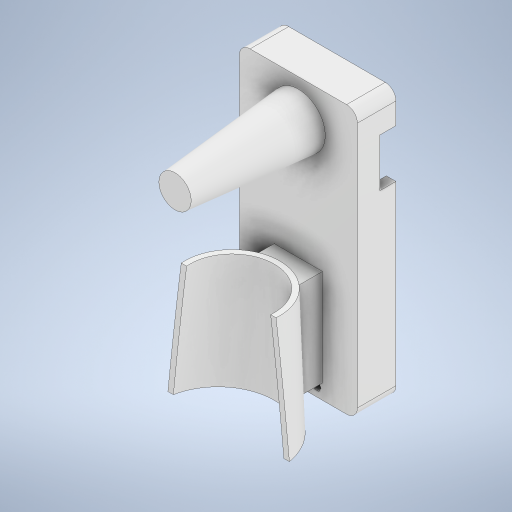
# Autodesk Inventor part: hand_rest_v4
Saved by Autodesk Inventor 2024 (Build 280153000, 153)
## iProperties
Created: 2023-07-30
Part Number: hand_rest_v4
Material: ABS Plastic
Document SubType Name: Modeling
Designer: Pintu
Density: 1.06 g/cm^3
Appearance: Smooth - White
Author: Pintu
Autodesk Inventor part; units mm, degrees
ref_plane "YZ Plane" through (0, 0, 0) normal (1, 0, 0) x (0, 1, 0)
ref_plane "XY Plane" through (0, 0, 0) normal (0, 0, 1) x (1, 0, 0)
sketch "Sketch1" plane through (0, 0, 0) normal (0, 0, 1) x (1, 0, 0)
  line L0 (-55, 125) -> (55, 125)
  line L1 (55, 125) -> (55, -125)
  line L2 (55, -125) -> (-55, -125)
  line L3 (-55, -125) -> (-55, 125)
  line L4 (-55, 125) -> (55, -125) construction
  line L5 (55, 125) -> (-55, -125) construction
  point P0 (0, 0)
  dimension "d0" = 110
  dimension "d1" = 250
  constraints: 12 end point, 2 midpoint, 2 parallel, 1 horizontal, 1 perpendicular
  measures "d0" distance of L1.end L2.end
  measures "d1" distance of L0.end L1.end
extrude "Extrusion1" add sketch "Sketch1" along normal blind 6
fillet "Fillet1" radius 10 4 edges at (-55, 125, 3) (55, 125, 3) (-55, -125, 3) (55, -125, 3)
sketch "Sketch2" plane through (0, 0, 6) normal (0, 0, 1) x (1, 0, 0)
  line L0 (-45, -125) -> (45, -125) projected
  point P0 (0, 0)
  point P1 (0.0434, -121)
  dimension "d5" = 4
  measures "d5" distance from line of L0 point (0.043, -121)
hole "Hole1" at (0.0434, -121, 6) direction (0, 0, -1) diameter 3 end through all
sketch "Sketch4" plane through (0, 0, 0) normal (0, 1, 0) x (-1, 0, 0)
  line L0 (-1.5434, 6) -> (1.4566, 6) projected
  line L1 (-55, 6) -> (-45, 6) projected
  line L2 (-45, 6) -> (-55, 6) projected
  line L3 (-45, 6) -> (45, 6) projected
  line L4 (55, 6) -> (45, 6) projected
  line L5 (45, 6) -> (55, 6) projected
  line L6 (45, 6) -> (-45, 6) projected
  circle A0 centre (0, 66) radius 42.5
  circle A1 centre (0, 66) radius 37.5
  point P0 (0, 0)
  point P1 (0, 6)
  dimension "frontOuterDia" = 85
  dimension "d17" = 60
  dimension "frontInnerDia" = 75
  constraints: 2 centre point, 1 coincident, 1 midpoint
  measures "frontOuterDia" diameter of A0
  measures "d17" distance of point (0, 6) A0.centre
  measures "frontInnerDia" diameter of A1
sketch "Sketch3" plane through (-45, -125, 0) normal (0, -1, 0) x (1, 0, 0)
  line L0 (0, 6) -> (90, 6) projected
  circle A0 centre (45, 81) radius 57.5
  circle A1 centre (45, 81) radius 52.5
  point P0 (45, 0)
  point P1 (45, 6)
  dimension "outerDia" = 115
  dimension "restHeight" = 75
  dimension "innerRearDia" = 105
  constraints: 2 centre point, 1 coincident, 1 midpoint
  measures "outerDia" diameter of A0
  measures "restHeight" distance of point (45, 6) A0.centre
  measures "innerRearDia" diameter of A1
loft "Loft1" add profiles "Sketch3", "Sketch4" contours A0 | A1 / A0 | A1
loft "Loft2" cut profiles "Sketch3", "Sketch4" contours A1 / A1
sketch "Sketch5" plane through (0, 0, 6) normal (0, 0, 1) x (1, 0, 0)
  line L0 (-22.5, -21) -> (22.5, -21)
  line L1 (22.5, -21) -> (22.5, -111)
  line L2 (22.5, -111) -> (-22.5, -111)
  line L3 (-22.5, -111) -> (-22.5, -21)
  line L4 (-22.5, -21) -> (22.5, -111) construction
  line L5 (22.5, -21) -> (-22.5, -111) construction
  line L6 (-45, -125) -> (45, -125) projected
  point P0 (0, 0)
  point P1 (0, -66)
  dimension "d27" = 45
  dimension "d28" = 90
  dimension "d142" = 14
  constraints: 12 end point, 2 midpoint, 2 parallel, 1 horizontal, 1 perpendicular
  measures "d27" distance of L1.end L2.end
  measures "d28" distance of L0.end L1.end
  measures "d142" distance between parallel lines of L6 L2
extrude "Extrusion2" add sketch "Sketch5" along normal blind 22
sketch "Sketch6" plane through (0, 0, 6) normal (0, 0, 1) x (1, 0, 0)
  circle A0 centre (0, 90) radius 25
  line L0 (45, 125) -> (-45, 125) projected
  line L1 (55, -115) -> (55, 115) projected
  point P0 (0, 0)
  dimension "d34" = 50
  dimension "d35" = 35
  dimension "d36" = 55
  constraints: 1 centre point
  measures "d34" diameter of A0
  measures "d35" distance from line of L0 A0.centre
  measures "d36" distance from line of L1 A0.centre
ref_plane "Work Plane3" through (0, 0, 121) normal (0, 0, 1) x (1, 0, 0)
sketch "Sketch7" plane through (0, 0, 121) normal (0, 0, 1) x (1, 0, 0)
  line L0 (45, 125) -> (-45, 125) projected
  circle A0 centre (0, 90) radius 15
  point P0 (0, 0)
  point P1 (0, 125)
  dimension "d38" = 30
  dimension "d39" = 35
  constraints: 1 centre point, 1 midpoint
  measures "d38" diameter of A0
  measures "d39" distance of point (0, 125) A0.centre
loft "Loft3" add profiles "Sketch6", "Sketch7"
ref_plane "Work Plane4" through (0, 0, 71) normal (0, 0, 1) x (1, 0, 0)
sketch "Sketch9" plane through (0, 0, 71) normal (0, 0, 1) x (1, 0, 0)
  line L0 (78.1064, 17.385) -> (-78.1064, 17.385)
  line L1 (-78.1064, 17.385) -> (-78.1064, -125.7261)
  line L2 (-78.1064, -125.7261) -> (78.1064, -125.7261)
  line L3 (78.1064, -125.7261) -> (78.1064, 17.385)
  line L4 (78.1064, 17.385) -> (-78.1064, -125.7261) construction
  line L5 (-78.1064, 17.385) -> (78.1064, -125.7261) construction
  point P0 (0, 0)
  point P1 (0, -54.1705)
  constraints: 12 end point, 2 midpoint, 2 parallel, 1 horizontal, 1 perpendicular
extrude "Extrusion4" cut sketch "Sketch9" along normal blind 100
ref_plane "Work Plane5" through (0, -15, 0) normal (0, 1, 0) x (-1, 0, 0)
sketch "Sketch19" plane through (0, -15, 0) normal (0, 1, 0) x (-1, 0, 0)
  point P0 (0, 0)
sketch "Sketch20" plane through (0, 0, 6) normal (0, 0, 1) x (1, 0, 0)
  line L0 (-80.5, -15) -> (80.5, -15) projected
  line L1 (55, -115) -> (55, 115) projected
  line L2 (-55, 115) -> (-55, -115) projected
  line L3 (55, -15) -> (-55, -15)
  line L4 (-55, -15) -> (-55, 0)
  line L5 (-55, 0) -> (55, 0)
  line L6 (55, 0) -> (55, -15)
  point P0 (0, 0)
  constraints: 8 end point, 2 parallel, 2 point on line, 1 horizontal, 1 midpoint, 1 perpendicular
extrude "Extrusion5" cut sketch "Sketch20" along normal blind 99.75
sketch "Sketch22" plane through (0, 0, 0) normal (0, 0, -1) x (-1, 0, 0)
  line L0 (55, 115) -> (55, -115) projected
  arc A0 (55, 115) -> (45, 125) centre (45, 115) ccw projected
  line L1 (-45, 125) -> (45, 125) projected
  arc A1 (-45, 125) -> (-55, 115) centre (-45, 115) ccw projected
  line L2 (-55, -115) -> (-55, 115) projected
  arc A2 (-55, -115) -> (-45, -125) centre (-45, -115) ccw projected
  line L3 (45, -125) -> (-45, -125) projected
  arc A3 (45, -125) -> (55, -115) centre (45, -115) ccw projected
  line L4 (46, -115) -> (46, 115)
  arc A4 (46, 115) -> (45, 116) centre (45, 115) ccw
  line L5 (45, 116) -> (-45, 116)
  arc A5 (-45, 116) -> (-46, 115) centre (-45, 115) ccw
  line L6 (-46, 115) -> (-46, -115)
  arc A6 (-46, -115) -> (-45, -116) centre (-45, -115) ccw
  line L7 (-45, -116) -> (45, -116)
  arc A7 (45, -116) -> (46, -115) centre (45, -115) ccw
  line L8 (-55, 95) -> (-37, 95)
  line L9 (-37, 95) -> (-37, 50)
  line L10 (-37, 50) -> (-55, 50)
  line L11 (-55, 50) -> (-55, 95)
  line L12 (0, -177.9853) -> (0, 178.4142) projected
  line L13 (22.5, -107) -> (-22.5, -107)
  line L14 (-22.5, -107) -> (-22.5, -125)
  line L15 (-22.5, -125) -> (22.5, -125)
  line L16 (22.5, -125) -> (22.5, -107)
  line L17 (22.5, -107) -> (-22.5, -125) construction
  line L18 (-22.5, -107) -> (22.5, -125) construction
  line L19 (55, 95) -> (37, 95)
  line L20 (37, 95) -> (37, 50)
  line L21 (37, 50) -> (55, 50)
  line L22 (55, 50) -> (55, 95)
  point P0 (0, 0)
  point P1 (0, -116)
  point P2 (-46, 95)
  point P3 (46, 95)
  point P4 (-22.5, -116)
  point P5 (-46, 50)
  point P6 (-55, 50)
  point P7 (46, 50)
  point P8 (22.5, -116)
  dimension "d146" = 9
  dimension "d147" = 18
  dimension "d148" = 45
  dimension "d149" = 30
  dimension "d150" = 45
  dimension "d151" = 18
  dimension "d152" = 0
  dimension "d153" = 18
  dimension "d154" = 45
  dimension "d155" = 30
  constraints: 36 end point, 8 point on circle, 6 parallel, 4 centre point, 3 horizontal, 3 perpendicular, 3 point on line, 2 midpoint, 7 other
  measures "d146" distance between parallel lines of L0 L4
  measures "d147" distance of L9.end L10.end
  measures "d148" distance of L8.end L9.end
  measures "d149" distance between parallel lines of L1 L8
  measures "d150" distance of L15.end L14.end
  measures "d151" distance of L14.end L13.end
  measures "d152" distance between parallel lines of L3 L15
  measures "d153" distance of L21.end L20.end
  measures "d154" distance of L20.end L19.end
  measures "d155" distance between parallel lines of L1 L19
extrude "Extrusion6" add sketch "Sketch22" along normal blind 30 contours L0 L19 L4 A4 L5 L12 L1 A0 | L0 A3 L3 L16 L7 A7 L4 L21 | L12 L5 A5 L6 L8 L2 A1 L1 | L10 L6 A6 L7 L14 L3 A2 L2
sketch "Sketch26" plane through (0, 0, 0) normal (0, 0, -1) x (-1, 0, 0)
  line L0 (-55, 115) -> (-55, 95) projected
  line L1 (-55, 95) -> (-46, 95) projected
  line L2 (-46, 95) -> (-46, 115) projected
  arc A0 (-45, 116) -> (-46, 115) centre (-45, 115) ccw projected
  line L3 (-45, 116) -> (45, 116) projected
  arc A1 (46, 115) -> (45, 116) centre (45, 115) ccw projected
  line L4 (46, 115) -> (46, 95) projected
  line L5 (46, 95) -> (55, 95) projected
  line L6 (55, 95) -> (55, 115) projected
  arc A2 (55, 115) -> (45, 125) centre (45, 115) ccw projected
  line L7 (45, 125) -> (-45, 125) projected
  arc A3 (-45, 125) -> (-55, 115) centre (-45, 115) ccw projected
  line L8 (46, 50) -> (46, -115) projected
  line L9 (55, -115) -> (55, 50) projected
  line L10 (55, 50) -> (46, 50) projected
  line L11 (46, 50) -> (46, -115) projected
  arc A4 (45, -116) -> (46, -115) centre (45, -115) ccw projected
  line L12 (45, -116) -> (22.5, -116) projected
  line L13 (22.5, -116) -> (22.5, -125) projected
  line L14 (22.5, -125) -> (45, -125) projected
  arc A5 (45, -125) -> (55, -115) centre (45, -115) ccw projected
  line L15 (-45, -125) -> (-22.5, -125) projected
  line L16 (-22.5, -125) -> (-22.5, -116) projected
  line L17 (-22.5, -116) -> (-45, -116) projected
  arc A6 (-46, -115) -> (-45, -116) centre (-45, -115) ccw projected
  line L18 (-46, -115) -> (-46, 50) projected
  line L19 (-46, 50) -> (-55, 50) projected
  line L20 (-55, 50) -> (-55, -115) projected
  arc A7 (-55, -115) -> (-45, -125) centre (-45, -115) ccw projected
  line L21 (-55, 95) -> (-37, 95)
  line L22 (-37, 95) -> (-37, 50)
  line L23 (-37, 50) -> (-55, 50)
  line L24 (-55, 50) -> (-55, 95)
  line L25 (-46, 50) -> (-55, 50) projected
  point P0 (0, 0)
  dimension "d168" = 18
  constraints: 8 end point, 2 parallel, 1 collinear, 1 horizontal, 1 perpendicular
  measures "d168" distance of L22.end L23.end
extrude "Extrusion8" add sketch "Sketch26" along normal blind 15 contours L1 L21 L22 L23 L19 L24
ref_plane "Work Plane6" through (46, 49, 0) normal (-1, 0, 0) x (0, 0, 1)
sketch "Sketch29" plane through (46, 49, 0) normal (-1, 0, 0) x (0, 0, 1)
  line L0 (-15, 46) -> (-15, 1) projected
  circle A0 centre (-15, 23.5) radius 11.5
  point P0 (0, -49)
  dimension "d171" = 23
  constraints: 1 centre point, 1 midpoint
  measures "d171" diameter of A0
extrude "Extrusion9" cut sketch "Sketch29" along normal mid plane 7
sketch "Sketch30" plane through (0, 0, 0) normal (0, 0, -1) x (-1, 0, 0)
  line L0 (-55, 115) -> (-55, 95) projected
  line L1 (-55, 95) -> (-46, 95) projected
  line L2 (-46, 95) -> (-46, 115) projected
  arc A0 (-45, 116) -> (-46, 115) centre (-45, 115) ccw projected
  line L3 (-45, 116) -> (45, 116) projected
  arc A1 (46, 115) -> (45, 116) centre (45, 115) ccw projected
  line L4 (46, 115) -> (46, 95) projected
  line L5 (46, 95) -> (55, 95) projected
  line L6 (55, 95) -> (55, 115) projected
  arc A2 (55, 115) -> (45, 125) centre (45, 115) ccw projected
  line L7 (45, 125) -> (-45, 125) projected
  arc A3 (-45, 125) -> (-55, 115) centre (-45, 115) ccw projected
  line L8 (55, -115) -> (55, 50) projected
  line L9 (55, 50) -> (46, 50) projected
  line L10 (46, 50) -> (46, -115) projected
  arc A4 (45, -116) -> (46, -115) centre (45, -115) ccw projected
  line L11 (45, -116) -> (22.5, -116) projected
  line L12 (22.5, -116) -> (22.5, -125) projected
  line L13 (22.5, -125) -> (45, -125) projected
  arc A5 (45, -125) -> (55, -115) centre (45, -115) ccw projected
  line L14 (-45, -125) -> (-22.5, -125) projected
  line L15 (-22.5, -125) -> (-22.5, -116) projected
  line L16 (-22.5, -116) -> (-45, -116) projected
  arc A6 (-46, -115) -> (-45, -116) centre (-45, -115) ccw projected
  line L17 (-46, -115) -> (-46, 50) projected
  line L18 (-46, 50) -> (-55, 50) projected
  line L19 (-55, 50) -> (-55, -115) projected
  arc A7 (-55, -115) -> (-45, -125) centre (-45, -115) ccw projected
  line L20 (55, 95) -> (55, 50) projected
  line L21 (55, 95) -> (37, 95)
  line L22 (37, 95) -> (37, 50)
  line L23 (37, 50) -> (55, 50)
  line L24 (55, 50) -> (55, 95)
  line L25 (-22.5, -125) -> (22.5, -125)
  line L26 (22.5, -125) -> (22.5, -107)
  line L27 (22.5, -107) -> (-22.5, -107)
  line L28 (-22.5, -107) -> (-22.5, -125)
  point P0 (0, 0)
  dimension "d174" = 18
  dimension "d175" = 18
  constraints: 16 end point, 4 parallel, 2 horizontal, 2 perpendicular, 1 point on line
  measures "d174" distance between parallel lines of L20 L22
  measures "d175" distance of L26.end L25.end
extrude "Extrusion10" add sketch "Sketch30" along normal blind 15 contours L20 L9 L23 L22 L21 L5 | L25 L15 L28 L27 L26 L12
ref_plane "Work Plane7" through (-46, -115, 6) normal (-1, 0, 0) x (0, 0, 1)
sketch "Sketch31" plane through (-46, -115, 6) normal (-1, 0, 0) x (0, 0, 1)
  line L0 (-21, 176) -> (-21, 199) projected
  circle A0 centre (-21, 187.5) radius 11.5
  point P0 (-6, 115)
  dimension "d178" = 23
  constraints: 1 centre point, 1 midpoint
  measures "d178" diameter of A0
extrude "Extrusion11" cut sketch "Sketch31" along normal mid plane 7
ref_plane "Work Plane9" through (-22.5, -116, 0) normal (0, 1, 0) x (1, 0, 0)
sketch "Sketch33" plane through (-22.5, -116, 0) normal (0, 1, 0) x (1, 0, 0)
  line L0 (45, 15) -> (0, 15) projected
  circle A0 centre (22.5, 15) radius 11.5
  point P0 (22.5, 0)
  dimension "d182" = 23
  constraints: 1 centre point, 1 midpoint
  measures "d182" diameter of A0
extrude "Extrusion12" cut sketch "Sketch33" along normal mid plane 7
fillet "Fillet15" radius 3 6 edges at (37, 50, -7.5) (37, 95, -7.5) (-37, 95, -7.5) (-37, 50, -7.5) (22.5, -107, -7.5) (-22.5, -107, -7.5) inverted yes
fillet "Fillet16" radius 2 12 edges at (19.5, -107, -7.5) (22.5, -110, -7.5) (-19.5, -107, -7.5) (-22.5, -110, -7.5) (37, 53, -7.5) (40, 50, -7.5) (37, 92, -7.5) (40, 95, -7.5) (-37, 92, -7.5) (-40, 95, -7.5) (-37, 53, -7.5) (-40, 50, -7.5)
sketch "Sketch45" plane through (0, 0, -15) normal (0, 0, -1) x (-1, 0, 0)
  line L0 (11.5, -112.5) -> (11.5, -119.5) projected
  line L1 (-22.5, -125) -> (22.5, -125) projected
  point P0 (0, 0)
  point P1 (17, -116)
  dimension "d236" = 5.5
  dimension "d237" = 9
  measures "d236" distance from line of L0 point (17, -116)
  measures "d237" distance from line of L1 point (17, -116)
hole "Hole12" at (-17, -116, -15) direction (0, 0, 1) diameter 4 depth 25 tip angle 118
sketch "Sketch46" plane through (0, 0, -15) normal (0, 0, -1) x (-1, 0, 0)
  line L0 (-11.5, -119.5) -> (-11.5, -112.5) projected
  line L1 (-22.5, -125) -> (22.5, -125) projected
  point P0 (0, 0)
  point P1 (-17, -116)
  dimension "d245" = 5.5
  dimension "d246" = 9
  measures "d245" distance from line of L0 point (-17, -116)
  measures "d246" distance from line of L1 point (-17, -116)
hole "Hole13" at (17, -116, -15) direction (0, 0, 1) diameter 4 depth 25 tip angle 118
sketch "Sketch47" plane through (0, 0, 6) normal (0, 0, 1) x (1, 0, 0)
  circle A0 centre (17, -116) radius 2 projected
  circle A1 centre (-17, -116) radius 2 projected
  line L0 (-11.5, -119.5) -> (11.5, -119.5) projected
  line L1 (11.5, -119.5) -> (11.5, -112.5) projected
  line L2 (11.5, -112.5) -> (-11.5, -112.5) projected
  line L3 (-11.5, -112.5) -> (-11.5, -119.5) projected
  arc A2 (-21.3, -109.7495) -> (-22.5, -111.5826) centre (-20.5, -111.5826) ccw projected
  arc A3 (-21.3, -109.7495) -> (-19.7505, -108.2) centre (-22.5, -107) ccw projected
  arc A4 (-17.9174, -107) -> (-19.7505, -108.2) centre (-17.9174, -109) ccw projected
  line L4 (-17.9174, -107) -> (17.9174, -107) projected
  arc A5 (19.7505, -108.2) -> (17.9174, -107) centre (17.9174, -109) ccw projected
  arc A6 (19.7505, -108.2) -> (21.3, -109.7495) centre (22.5, -107) ccw projected
  arc A7 (22.5, -111.5826) -> (21.3, -109.7495) centre (20.5, -111.5826) ccw projected
  line L5 (22.5, -111.5826) -> (22.5, -116) projected
  line L6 (22.5, -125) -> (22.5, -116) projected
  line L7 (22.5, -125) -> (-22.5, -125) projected
  line L8 (-22.5, -116) -> (-22.5, -125) projected
  line L9 (-22.5, -116) -> (-22.5, -111.5826) projected
  line L10 (-14.9215, -119.6) -> (-19.0785, -119.6)
  line L11 (-19.0785, -119.6) -> (-21.1569, -116)
  line L12 (-21.1569, -116) -> (-19.0785, -112.4)
  line L13 (-19.0785, -112.4) -> (-14.9215, -112.4)
  line L14 (-14.9215, -112.4) -> (-12.8431, -116)
  line L15 (-12.8431, -116) -> (-14.9215, -119.6)
  line L16 (19.0785, -119.6) -> (14.9215, -119.6)
  line L17 (14.9215, -119.6) -> (12.8431, -116)
  line L18 (12.8431, -116) -> (14.9215, -112.4)
  line L19 (14.9215, -112.4) -> (19.0785, -112.4)
  line L20 (19.0785, -112.4) -> (21.1569, -116)
  line L21 (21.1569, -116) -> (19.0785, -119.6)
  point P0 (0, 0)
  point P1 (-17, -119.6)
  point P2 (-17, -112.4)
  dimension "d254" = 7.2
  constraints: 24 end point, 2 coincident, 2 midpoint, 2 parallel, 1 point on line, 26 other
  measures "d254" distance of point (-17, -119.6) point (-17, -112.4)
extrude "Extrusion20" cut sketch "Sketch47" against normal blind 10 contours A0 | A1 | L10 L11 L12 L13 L14 L15 | L16 L17 L18 L19 L20 L21
body "Solid1"
